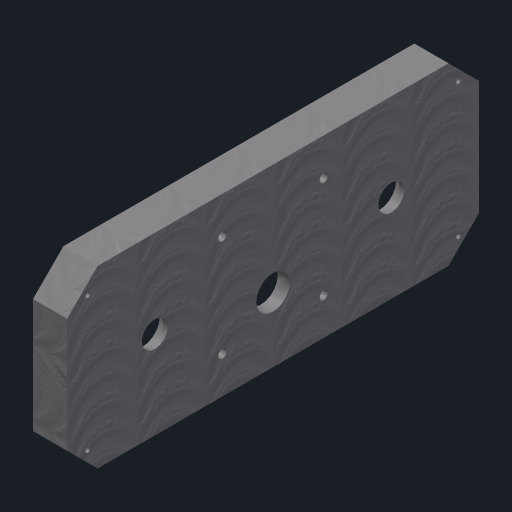
# Autodesk Inventor part: CAJA
Saved by Autodesk Inventor 2024.3 (Build 283343000, 343)
## iProperties
Created: 2024-06-29
Part Number: CAJA
Material: Steel, Mild, Welded
Document SubType Name: Modeling
Designer: Niler
Density: 7.85 g/cm^3
Appearance: Weld - Steel Mild
Author: Niler
Autodesk Inventor part; units mm, degrees
ref_plane "YZ Plane" through (0, 0, 0) normal (1, 0, 0) x (0, 1, 0)
ref_plane "XZ Plane" through (0, 0, 0) normal (0, 1, 0) x (-1, 0, 0)
ref_plane "XY Plane" through (0, 0, 0) normal (0, 0, 1) x (1, 0, 0)
sketch "Sketch1" plane through (0, 0, 0) normal (1, 0, 0) x (0, 1, 0)
  line L0 (-57.5, 135) -> (57.5, 135)
  line L1 (57.5, 135) -> (57.5, -135)
  line L2 (57.5, -135) -> (-57.5, -135)
  line L3 (-57.5, -135) -> (-57.5, 135)
  line L4 (-57.5, 135) -> (57.5, -135) construction
  line L5 (57.5, 135) -> (-57.5, -135) construction
  circle A0 centre (0, 77.5) radius 3.925
  circle A1 centre (0, -77.5) radius 3.925
  circle A2 centre (-15, 0) radius 5
  line L6 (0, 77.5) -> (0, -77.5) construction
  line L7 (50.5, -128) -> (50.5, 128)
  line L8 (50.5, 128) -> (-50.5, 128)
  line L9 (-50.5, 128) -> (-50.5, -128)
  line L10 (-50.5, -128) -> (50.5, -128)
  point P0 (0, 0)
  dimension "d0" = 155
  dimension "d1" = 7.85
  dimension "d2" = 270
  dimension "d3" = 115
  dimension "d4" = 7
  dimension "d35" = 10
  dimension "d36" = 15
  constraints: 22 end point, 4 parallel, 3 centre point, 3 midpoint, 2 perpendicular, 1 equal radius, 1 horizontal, 1 horizontal alignment, 1 vertical, 1 vertical alignment, 3 other
  measures "d0" distance of L6.end L6.start
  measures "d1" diameter of A0
  measures "d2" distance between parallel lines of L2 L0
  measures "d3" distance of L0.start L0.end
  measures "d4" distance between parallel lines of L1 L7
  measures "d35" diameter of A2
  measures "d36" distance of A2.centre point (0, 0)
extrude "Extrusion1" add sketch "Sketch1" along normal blind 8 contours L0 L1 L2 L3 | A0 | A1 | L10 L9 L8 L7
extrude "Extrusion2" add sketch "Sketch1" against normal blind 14.4 contours L0 L1 L2 L3
sketch "Sketch2" plane through (8, 0, 0) normal (1, 0, 0) x (0, 0, -1)
  line L0 (135, -57.5) -> (135, 57.5) projected
  line L1 (135, 57.5) -> (-135, 57.5) projected
  line L2 (-135, 57.5) -> (-135, -57.5) projected
  line L3 (-135, -57.5) -> (135, -57.5) projected
  line L4 (-33.234, -33.234) -> (33.234, -33.234) construction
  line L5 (33.234, -33.234) -> (33.234, 33.234) construction
  line L6 (33.234, 33.234) -> (-33.234, 33.234) construction
  line L7 (-33.234, 33.234) -> (-33.234, -33.234) construction
  line L8 (-33.234, -33.234) -> (33.234, 33.234) construction
  line L9 (33.234, -33.234) -> (-33.234, 33.234) construction
  circle A0 centre (0, 0) radius 47 construction
  circle A1 centre (33.234, 33.234) radius 2.75
  circle A2 centre (-33.234, 33.234) radius 2.75
  circle A3 centre (0, 0) radius 47 construction
  circle A4 centre (-33.234, -33.234) radius 2.75
  circle A5 centre (0, 0) radius 47 construction
  circle A6 centre (33.234, -33.234) radius 2.75
  circle A7 centre (0, 0) radius 47 construction
  point P0 (0, 0)
  point P1 (0, 0)
  dimension "d12" = 94
  dimension "d13" = 5.5
  dimension "d16" = 360
  constraints: 12 end point, 7 coincident, 4 centre point, 2 parallel, 2 perpendicular, 1 horizontal, 1 midpoint, 31 other
  measures "d13" diameter of A1
extrude "Extrusion3" cut sketch "Sketch2" against normal through all contours A1 | A2 | A4 | A6
sketch "Sketch3" plane through (0, 0, 0) normal (-1, 0, 0) x (0, 0, 1)
  circle A0 centre (33.234, -33.234) radius 2.75 projected
  circle A1 centre (33.234, 33.234) radius 2.75 projected
  circle A2 centre (-33.234, -33.234) radius 2.75 projected
  circle A3 centre (-33.234, 33.234) radius 2.75 projected
  line L0 (-128, -50.5) -> (128, -50.5) projected
  line L1 (128, -50.5) -> (128, 50.5) projected
  line L2 (128, 50.5) -> (-128, 50.5) projected
  line L3 (-128, 50.5) -> (-128, -50.5) projected
  circle A4 centre (0, -15) radius 5 projected
  circle A5 centre (-33.234, 33.234) radius 4.5
  circle A6 centre (33.234, 33.234) radius 2.75 projected
  circle A7 centre (33.234, 33.234) radius 4.5
  circle A8 centre (-33.234, -33.234) radius 4.5
  circle A9 centre (33.234, -33.234) radius 4.5
  point P0 (0, 0)
  dimension "d20" = 9
  constraints: 4 centre point, 4 coincident, 3 equal radius
  measures "d20" diameter of A5
extrude "Extrusion4" cut sketch "Sketch3" against normal blind 3 contours A0 | A1 | A2 | A3 | A5 | A7 | A8 | A9
sketch "Sketch4" plane through (8, 0, 0) normal (1, 0, 0) x (0, 0, -1)
  circle A0 centre (-33.234, -33.234) radius 2.75 projected
  circle A1 centre (-33.234, 33.234) radius 2.75 projected
  circle A2 centre (33.234, -33.234) radius 2.75 projected
  circle A3 centre (33.234, 33.234) radius 2.75 projected
  line L0 (135, -57.5) -> (135, 57.5) projected
  line L1 (135, 57.5) -> (-135, 57.5) projected
  line L2 (-135, 57.5) -> (-135, -57.5) projected
  line L3 (-135, -57.5) -> (135, -57.5) projected
  circle A4 centre (0, -15) radius 5 projected
  circle A5 centre (0, -15) radius 11
  point P0 (0, 0)
  dimension "d24" = 22
  constraints: 1 centre point, 1 coincident
  measures "d24" diameter of A5
extrude "Extrusion5" cut sketch "Sketch4" against normal through all contours A4 | A5
chamfer "Chamfer2" distance 20 angle 45 8 edges at (-7.2, 50.5, -128) (-7.2, -50.5, -128) (-7.2, -50.5, 128) (-7.2, 50.5, 128) (-3.2, 57.5, -135) (-3.2, -57.5, -135) (-3.2, -57.5, 135) (-3.2, 57.5, 135)
sketch "Sketch6" plane through (-14.4, 0, 0) normal (-1, 0, 0) x (0, 0, 1)
  line L0 (115, 57.5) -> (135, 37.5) projected
  line L1 (115, 57.5) -> (-115, 57.5) projected
  line L2 (-135, 37.5) -> (-115, 57.5) projected
  line L3 (-135, 37.5) -> (-135, -37.5) projected
  line L4 (-115, -57.5) -> (-135, -37.5) projected
  line L5 (-115, -57.5) -> (115, -57.5) projected
  line L6 (135, -37.5) -> (115, -57.5) projected
  line L7 (135, -37.5) -> (135, 37.5) projected
  line L8 (-128, -30.5) -> (-128, 30.5) projected
  line L9 (-108, 50.5) -> (-128, 30.5) projected
  line L10 (-108, 50.5) -> (108, 50.5) projected
  line L11 (128, 30.5) -> (108, 50.5) projected
  line L12 (128, 30.5) -> (128, -30.5) projected
  line L13 (108, -50.5) -> (128, -30.5) projected
  line L14 (108, -50.5) -> (-108, -50.5) projected
  line L15 (-128, -30.5) -> (-108, -50.5) projected
  line L16 (121.5, -44) -> (-121.5, -44)
  line L17 (-121.5, -44) -> (-121.5, 44)
  line L18 (-121.5, 44) -> (121.5, 44)
  line L19 (121.5, 44) -> (121.5, -44)
  circle A0 centre (0, 0) radius 10.3
  line L20 (121.5, -44) -> (-121.5, 44) construction
  line L21 (-121.5, -44) -> (121.5, 44) construction
  circle A1 centre (-121.5, 44) radius 1.5
  circle A2 centre (-121.5, -44) radius 1.5
  circle A3 centre (121.5, -44) radius 1.5
  circle A4 centre (121.5, 44) radius 1.5
  line L22 (-125, 47.5) -> (-118, 40.5)
  dimension "d32" = 3
  constraints: 14 end point, 5 centre point, 5 coincident, 5 midpoint, 3 equal radius, 2 parallel, 1 horizontal, 1 perpendicular
  measures "d32" diameter of A1
extrude "Extrusion7" cut sketch "Sketch6" against normal through all contours A2 L16 L17 | L17 L16 A2 | A1 L22 L17 | L17 L22 A1 | L22 L18 A1 | L22 A1 L18 | A3 L19 L16 | L16 L19 A3 | A4 L19 L18 | L18 L19 A4
sketch "Sketch12" plane through (0, 0, 0) normal (-1, 0, 0) x (0, 0, 1)
  circle A0 centre (-77.5, 0) radius 3.925 projected
  circle A1 centre (77.5, 0) radius 3.925 projected
  circle A2 centre (-77.5, 0) radius 11.15
  circle A3 centre (77.5, 0) radius 11.15
  point P0 (0, 0)
  dimension "d61" = 22.3
  constraints: 2 centre point, 2 coincident, 1 equal radius
  measures "d61" diameter of A2
extrude "Extrusion13" cut sketch "Sketch12" against normal blind 5 contours A0 | A1 | A2 | A3
sketch "Sketch13" plane through (5, 0, -77.5) normal (-1, 0, 0) x (0, 0, 1)
  circle A0 centre (0, 0) radius 11.15 projected
  circle A1 centre (155, 0) radius 11.15 projected
  circle A2 centre (0, 0) radius 8.5
  circle A3 centre (155, 0) radius 8.5
  point P0 (77.5, 0)
  dimension "d64" = 17
  dimension "d65" = 17
  constraints: 2 centre point, 2 coincident
  measures "d64" diameter of A2
  measures "d65" diameter of A3
extrude "Extrusion14" cut sketch "Sketch13" against normal through all contours A2 | A3
body "Solid1"
